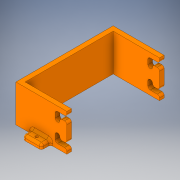
# Autodesk Inventor part: batery holder side opening
Saved by Autodesk Inventor 2019 (Build 230136000, 136)
## iProperties
Created: 2019-11-19
Part Number: batery holder side opening
Material: Generic
Document SubType Name: Modeling
Designer: User
Density: 1 g/cm^3
Appearance: Default(1)
Author: User
Autodesk Inventor part; units mm, degrees
ref_plane "YZ Plane" through (0, 0, 0) normal (1, 0, 0) x (0, 1, 0)
ref_plane "XZ Plane" through (0, 0, 0) normal (0, 1, 0) x (-1, 0, 0)
ref_plane "XY Plane" through (0, 0, 0) normal (0, 0, 1) x (1, 0, 0)
sketch "Sketch1" plane through (0, 0, 0) normal (0, 1, 0) x (-1, 0, 0)
  line L0 (0, 0) -> (63.5, 0)
  line L1 (63.5, 0) -> (63.5, -6.35)
  line L2 (63.5, -6.35) -> (0, -6.35)
  line L3 (0, -6.35) -> (0, 0)
  line L4 (63.5, 0) -> (69.85, 0)
  line L5 (69.85, 0) -> (69.85, -133.35)
  line L6 (69.85, -133.35) -> (63.5, -133.35)
  line L7 (63.5, -133.35) -> (63.5, 0)
  line L8 (69.85, -133.35) -> (0, -133.35)
  line L9 (0, -133.35) -> (0, -127)
  line L10 (0, -127) -> (69.85, -127)
  line L11 (69.85, -127) -> (69.85, -133.35)
  dimension "d0" = 6.35
  dimension "d1" = 6.35
  dimension "d2" = 6.35
  dimension "d3" = 120.65
  dimension "d4" = 63.5
  constraints: 24 end point, 6 parallel, 3 horizontal, 3 perpendicular, 1 point on line
  measures "d0" distance between parallel lines of L0 L2
  measures "d1" distance of L8.end L9.end
  measures "d2" distance of L5.end L6.end
  measures "d3" distance between parallel lines of L10 L2
  measures "d4" distance between parallel lines of L9 L7
extrude "Extrusion1" add sketch "Sketch1" along normal blind 50.8
sketch "Sketch6" plane through (-69.85, 0, 0) normal (0, 0, 1) x (1, 0, 0)
  line L0 (69.85, 0) -> (69.85, 50.8) projected
  line L1 (69.85, 12.7) -> (60.325, 12.7)
  line L2 (60.325, 12.7) -> (60.325, 6.35)
  line L3 (60.325, 6.35) -> (69.85, 6.35)
  line L4 (69.85, 6.35) -> (69.85, 12.7)
  line L5 (60.325, 6.35) -> (53.975, 6.35)
  line L6 (53.975, 6.35) -> (53.975, 19.05)
  line L7 (53.975, 19.05) -> (60.325, 19.05)
  line L8 (60.325, 19.05) -> (60.325, 6.35)
  line L9 (69.85, 44.45) -> (60.325, 44.45)
  line L10 (60.325, 44.45) -> (60.325, 38.1)
  line L11 (60.325, 38.1) -> (69.85, 38.1)
  line L12 (69.85, 38.1) -> (69.85, 44.45)
  line L13 (60.325, 44.45) -> (53.975, 44.45)
  line L14 (53.975, 44.45) -> (53.975, 31.75)
  line L15 (53.975, 31.75) -> (60.325, 31.75)
  line L16 (60.325, 31.75) -> (60.325, 44.45)
  line L17 (0, 50.8) -> (69.85, 50.8) projected
  line L18 (0, 0) -> (69.85, 0) projected
  dimension "d102" = 6.35
  dimension "d104" = 9.525
  dimension "d105" = 6.35
  dimension "d106" = 6.35
  dimension "d107" = 12.7
  dimension "d108" = 12.7
  dimension "d109" = 6.35
  dimension "d110" = 6.35
  constraints: 32 end point, 8 parallel, 4 horizontal, 4 perpendicular, 4 point on line
  measures "d102" distance between parallel lines of L11 L9
  measures "d104" distance between parallel lines of L2 L0
  measures "d105" distance between parallel lines of L3 L1
  measures "d106" distance between parallel lines of L8 L6
  measures "d107" distance between parallel lines of L5 L7
  measures "d108" distance between parallel lines of L15 L13
  measures "d109" distance between parallel lines of L9 L17
  measures "d110" distance between parallel lines of L18 L5
extrude "Extrusion6" cut sketch "Sketch6" against normal blind 152.4
fillet "Fillet4" radius 3.175 16 edges at (-15.875, 31.75, -3.175) (-15.875, 6.35, -3.175) (-15.875, 6.35, -130.175) (-15.875, 19.05, -3.175) (-9.525, 19.05, -3.175) (-15.875, 44.45, -3.175) (-15.875, 44.45, -130.175) (-9.525, 31.75, -3.175) (-9.525, 38.1, -3.175) (-9.525, 12.7, -3.175) (-15.875, 31.75, -130.175) (-9.525, 31.75, -130.175) (-9.525, 38.1, -130.175) (-15.875, 19.05, -130.175) (-9.525, 19.05, -130.175) (-9.525, 12.7, -130.175)
fillet "Fillet5" radius 3.175 8 edges at (0, 44.45, -3.175) (0, 38.1, -3.175) (0, 12.7, -3.175) (0, 6.35, -3.175) (0, 6.35, -130.175) (0, 12.7, -130.175) (0, 38.1, -130.175) (0, 44.45, -130.175)
sketch "Sketch7" plane through (-69.85, 0, 0) normal (0, 0, 1) x (1, 0, 0)
  line L0 (22.225, 0) -> (47.625, 0)
  line L1 (47.625, 0) -> (47.625, 6.35)
  line L2 (47.625, 6.35) -> (22.225, 6.35)
  line L3 (22.225, 6.35) -> (22.225, 0)
  line L4 (0, 0) -> (69.85, 0) projected
  line L5 (69.85, 15.875) -> (69.85, 34.925) projected
  line L6 (0, 0) -> (0, 50.8) projected
  dimension "d116" = 6.35
  dimension "d117" = 25.4
  dimension "d118" = 0
  dimension "d119" = 69.85
  dimension "d120" = 22.225
  constraints: 8 end point, 2 parallel, 1 horizontal, 1 perpendicular
  measures "d116" distance of L2.end L0.start
  measures "d117" distance between parallel lines of L1 L3
  measures "d118" distance between parallel lines of L4 L0
  measures "d119" distance between parallel lines of L5 L6
  measures "d120" distance between parallel lines of L6 L3
extrude "Extrusion7" add sketch "Sketch7" along normal blind 12.7
sketch "Sketch8" plane through (0, 0, -133.35) normal (0, 0, -1) x (-1, 0, 0)
  line L0 (22.225, 0) -> (47.625, 0)
  line L1 (47.625, 0) -> (47.625, 6.35)
  line L2 (47.625, 6.35) -> (22.225, 6.35)
  line L3 (22.225, 6.35) -> (22.225, 0)
  line L4 (69.85, 0) -> (69.85, 50.8) projected
  line L5 (0, 15.875) -> (0, 34.925) projected
  line L6 (0, 0) -> (69.85, 0) projected
  dimension "d123" = 25.4
  dimension "d124" = 6.35
  dimension "d125" = 69.85
  dimension "d126" = 22.225
  dimension "d127" = 6.35
  constraints: 8 end point, 2 parallel, 1 horizontal, 1 perpendicular
  measures "d123" distance between parallel lines of L1 L3
  measures "d124" distance between parallel lines of L2 L0
  measures "d125" distance between parallel lines of L4 L5
  measures "d126" distance between parallel lines of L3 L5
  measures "d127" distance between parallel lines of L2 L6
extrude "Extrusion8" add sketch "Sketch8" along normal blind 12.7
fillet "Fillet6" radius 3.175 16 edges at (-22.225, 3.175, -133.35) (-34.925, 6.35, -133.35) (-47.625, 3.175, -133.35) (-47.625, 3.175, 0) (-34.925, 6.35, 0) (-34.925, 6.35, 12.7) (-47.625, 6.35, 6.35) (-22.225, 6.35, 6.35) (-22.225, 3.175, 0) (-47.625, 6.35, -139.7) (-22.225, 6.35, -139.7) (-34.925, 6.35, -146.05) (-22.225, 3.175, 12.7) (-47.625, 3.175, 12.7) (-47.625, 3.175, -146.05) (-22.225, 3.175, -146.05)
sketch "Sketch9" plane through (-44.45, 6.35, -142.875) normal (0, 1, 0) x (1, 0, 0)
  line L0 (-25.4, -142.875) -> (44.45, -142.875) projected
  line L1 (22.225, -152.4) -> (22.225, -146.05) projected
  line L2 (44.45, -9.525) -> (-25.4, -9.525) projected
  line L3 (22.225, -6.35) -> (22.225, 0) projected
  point P0 (9.525, -149.225)
  point P1 (9.525, -3.175)
  dimension "d131" = 6.35
  dimension "d132" = 12.7
  dimension "d133" = 6.35
  dimension "d134" = 12.7
  measures "d131" distance from line of point (9.525, -149.225) L0
  measures "d132" distance from line of L1 point (9.525, -149.225)
  measures "d133" distance from line of point (9.525, -3.175) L2
  measures "d134" distance from line of L3 point (9.525, -3.175)
hole "Hole2" at (-34.925, 6.35, 6.35) at (-34.925, 6.35, -139.7) direction (0, -1, 0) diameter 3.81 end through all clearance for "Flat Head Machine Screw (82)" size "#6" standard "Ansi Unified Screw Threads"
equation "\"d0\" = d2"
equation "\"d2\" = d1"
equation "\"d105\" = d102"
equation "\"d106\" = d105"
equation "\"d108\" = d107"
equation "\"d109\" = d110"
equation "\"d120\" = -0.5 * d117 + 0.5 * d119"
equation "\"d126\" = -0.5 * d123 + 0.5 * d125"
equation "\"d127\" = d124"
body "Solid1"
